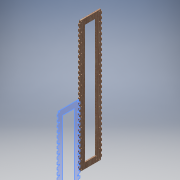
# Autodesk Inventor part: ArmTo
Saved by Autodesk Inventor 2019 (Build 230136000, 136)
## iProperties
Created: 2019-01-14
Part Number: ArmTo
Material: Wood (Birch)
Document SubType Name: Modeling
Designer: nxgam
Density: 0.55 g/cm^3
Appearance: Birch - Natural Polished
Author: nxgam
Autodesk Inventor part; units mm, degrees
ref_plane "YZ Plane" through (0, 0, 0) normal (1, 0, 0) x (0, 1, 0)
ref_plane "XZ Plane" through (0, 0, 0) normal (0, 1, 0) x (-1, 0, 0)
ref_plane "XY Plane" through (0, 0, 0) normal (0, 0, 1) x (1, 0, 0)
sketch "Sketch1" plane through (0, 0, 0) normal (1, 0, 0) x (0, 1, 0)
  line L0 (0, 50.8) -> (579.12, 50.8)
  line L1 (579.12, 50.8) -> (579.12, -50.8)
  line L2 (579.12, -50.8) -> (0, -50.8)
  line L3 (0, -50.8) -> (0, 50.8)
  point P0 (0, 0)
  point P1 (0, 0)
  dimension "d0" = 579.12
  dimension "d1" = 101.6
  constraints: 8 end point, 2 parallel, 1 coincident, 1 horizontal, 1 midpoint, 1 perpendicular, 1 other
  measures "d0" distance of L1.end L2.end
  measures "d1" distance of L0.end L1.end
extrude "Extrusion1" add sketch "Sketch1" along normal blind 5.08
sketch "Sketch2" plane through (5.08, 0, 0) normal (1, 0, 0) x (0, 0, -1)
  line L0 (-50.8, 579.12) -> (-50.8, 0) projected
  line L1 (-50.8, 0) -> (50.8, 0) projected
  line L2 (50.8, 0) -> (50.8, 579.12) projected
  line L3 (50.8, 579.12) -> (-50.8, 579.12) projected
  line L4 (-25.4, 553.72) -> (-25.4, 25.4)
  line L5 (-25.4, 25.4) -> (25.4, 25.4)
  line L6 (25.4, 25.4) -> (25.4, 553.72)
  line L7 (25.4, 553.72) -> (-25.4, 553.72)
  point P0 (0, 0)
  dimension "d4" = 50.8
  constraints: 8 end point, 3 other
  measures "d4" distance between parallel lines of L4 L6
extrude "Extrusion2" cut sketch "Sketch2" against normal blind 5.08 contours L7 L6 L5 L4
sketch "Sketch3" plane through (5.08, 0, 0) normal (1, 0, 0) x (0, 0, -1)
  circle A0 centre (-40.64, 45.72) radius 2 projected
  circle A1 centre (40.64, 5.08) radius 2 projected
  circle A2 centre (-40.64, 5.08) radius 2 projected
  circle A3 centre (40.64, 45.72) radius 2 projected
  line L0 (-42.545, 0) -> (42.545, 0) projected
  line L1 (45.72, 3.175) -> (45.72, 62.865) projected
  line L2 (42.545, 66.04) -> (38.735, 66.04) projected
  line L3 (35.56, 62.865) -> (35.56, 10.16) projected
  line L4 (35.56, 10.16) -> (-35.56, 10.16) projected
  line L5 (-35.56, 10.16) -> (-35.56, 62.865) projected
  line L6 (-38.735, 66.04) -> (-42.545, 66.04) projected
  line L7 (-45.72, 62.865) -> (-45.72, 3.175) projected
  arc A4 (-45.72, 3.175) -> (-42.545, 0) centre (-42.545, 3.175) ccw projected
  arc A5 (42.545, 0) -> (45.72, 3.175) centre (42.545, 3.175) ccw projected
  arc A6 (45.72, 62.865) -> (42.545, 66.04) centre (42.545, 62.865) ccw projected
  arc A7 (38.735, 66.04) -> (35.56, 62.865) centre (38.735, 62.865) ccw projected
  arc A8 (-35.56, 62.865) -> (-38.735, 66.04) centre (-38.735, 62.865) ccw projected
  arc A9 (-42.545, 66.04) -> (-45.72, 62.865) centre (-42.545, 62.865) ccw projected
  point P0 (0, 0)
  point P1 (-40.64, 45.72)
  point P2 (40.64, 5.08)
  point P3 (40.64, 45.72)
  point P4 (-40.64, 86.36)
  point P5 (40.64, 86.36)
  point P6 (-40.64, 127)
  point P7 (40.64, 127)
  point P8 (-40.64, 167.64)
  point P9 (40.64, 167.64)
  point P10 (-40.64, 208.28)
  point P11 (40.64, 208.28)
  point P12 (-40.64, 248.92)
  point P13 (40.64, 248.92)
  point P14 (-40.64, 289.56)
  point P15 (40.64, 289.56)
  point P16 (-40.64, 330.2)
  point P17 (40.64, 330.2)
  point P18 (-40.64, 370.84)
  point P19 (40.64, 370.84)
  point P20 (-40.64, 411.48)
  point P21 (40.64, 411.48)
  point P22 (-40.64, 452.12)
  point P23 (40.64, 452.12)
  point P24 (-40.64, 492.76)
  point P25 (40.64, 492.76)
  point P26 (-40.64, 533.4)
  point P27 (40.64, 533.4)
  point P28 (-40.64, 574.04)
  point P29 (40.64, 574.04)
  dimension "d9" = 40.64
  constraints: 4 coincident, 1 vertical, 26 other
  measures "d9" distance of point (-40.64, 45.72) point (-40.64, 86.36)
hole "Hole1" at (5.08, 5.08, 40.64) at (5.08, 45.72, 40.64) at (5.08, 5.08, -40.64) at (5.08, 45.72, -40.64) at (5.08, 86.36, 40.64) at (5.08, 86.36, -40.64) at (5.08, 127, 40.64) at (5.08, 127, -40.64) at (5.08, 167.64, 40.64) at (5.08, 167.64, -40.64) at (5.08, 208.28, 40.64) at (5.08, 208.28, -40.64) at (5.08, 248.92, 40.64) at (5.08, 248.92, -40.64) at (5.08, 289.56, 40.64) at (5.08, 289.56, -40.64) at (5.08, 330.2, 40.64) at (5.08, 330.2, -40.64) at (5.08, 370.84, 40.64) at (5.08, 370.84, -40.64) at (5.08, 411.48, 40.64) at (5.08, 411.48, -40.64) at (5.08, 452.12, 40.64) at (5.08, 452.12, -40.64) at (5.08, 492.76, 40.64) at (5.08, 492.76, -40.64) at (5.08, 533.4, 40.64) at (5.08, 533.4, -40.64) at (5.08, 574.04, 40.64) at (5.08, 574.04, -40.64) direction (-1, 0, 0) diameter 4 end through all
sketch "Sketch5" plane through (5.08, 0, 0) normal (1, 0, 0) x (0, 0, -1)
  circle A0 centre (-40.64, 574.04) radius 2 projected
  circle A1 centre (-40.64, 533.4) radius 2 projected
  circle A2 centre (-40.64, 492.76) radius 2 projected
  circle A3 centre (-40.64, 452.12) radius 2 projected
  circle A4 centre (-40.64, 411.48) radius 2 projected
  circle A5 centre (-40.64, 370.84) radius 2 projected
  circle A6 centre (-40.64, 330.2) radius 2 projected
  circle A7 centre (-40.64, 289.56) radius 2 projected
  circle A8 centre (-40.64, 248.92) radius 2 projected
  circle A9 centre (-40.64, 208.28) radius 2 projected
  circle A10 centre (-40.64, 167.64) radius 2 projected
  circle A11 centre (-40.64, 127) radius 2 projected
  circle A12 centre (-40.64, 86.36) radius 2 projected
  circle A13 centre (40.64, 5.08) radius 2 projected
  circle A14 centre (-40.64, 5.08) radius 2 projected
  circle A15 centre (-40.64, 45.72) radius 2 projected
  circle A16 centre (40.64, 45.72) radius 2 projected
  circle A17 centre (40.64, 86.36) radius 2 projected
  circle A18 centre (40.64, 127) radius 2 projected
  circle A19 centre (40.64, 167.64) radius 2 projected
  circle A20 centre (40.64, 208.28) radius 2 projected
  circle A21 centre (40.64, 248.92) radius 2 projected
  circle A22 centre (40.64, 289.56) radius 2 projected
  circle A23 centre (40.64, 330.2) radius 2 projected
  circle A24 centre (40.64, 370.84) radius 2 projected
  circle A25 centre (40.64, 411.48) radius 2 projected
  circle A26 centre (40.64, 452.12) radius 2 projected
  circle A27 centre (40.64, 492.76) radius 2 projected
  circle A28 centre (40.64, 533.4) radius 2 projected
  circle A29 centre (40.64, 574.04) radius 2 projected
  line L0 (25.4, 25.4) -> (-25.4, 25.4) projected
  line L1 (-25.4, 25.4) -> (-25.4, 553.72) projected
  line L2 (-25.4, 553.72) -> (25.4, 553.72) projected
  line L3 (25.4, 553.72) -> (25.4, 25.4) projected
  line L4 (-50.8, 579.12) -> (-50.8, 0) projected
  line L5 (-50.8, 0) -> (50.8, 0) projected
  line L6 (50.8, 0) -> (50.8, 579.12) projected
  line L7 (50.8, 579.12) -> (-50.8, 579.12) projected
  line L8 (-50.8, 579.12) -> (-45.72, 579.12)
  line L9 (-45.72, 579.12) -> (-45.72, 568.96)
  line L10 (-45.72, 568.96) -> (-50.8, 568.96)
  line L11 (-50.8, 568.96) -> (-50.8, 579.12)
  line L12 (-45.72, 558.8) -> (-45.72, 548.64)
  line L13 (-50.8, 548.64) -> (-50.8, 558.8)
  line L14 (-45.72, 548.64) -> (-50.8, 548.64)
  line L15 (-50.8, 558.8) -> (-45.72, 558.8)
  line L16 (-45.72, 538.48) -> (-45.72, 528.32)
  line L17 (-50.8, 528.32) -> (-50.8, 538.48)
  line L18 (-45.72, 528.32) -> (-50.8, 528.32)
  line L19 (-50.8, 538.48) -> (-45.72, 538.48)
  line L20 (-45.72, 518.16) -> (-45.72, 508)
  line L21 (-50.8, 508) -> (-50.8, 518.16)
  line L22 (-45.72, 508) -> (-50.8, 508)
  line L23 (-50.8, 518.16) -> (-45.72, 518.16)
  line L24 (-45.72, 497.84) -> (-45.72, 487.68)
  line L25 (-50.8, 487.68) -> (-50.8, 497.84)
  line L26 (-45.72, 487.68) -> (-50.8, 487.68)
  line L27 (-50.8, 497.84) -> (-45.72, 497.84)
  line L28 (-45.72, 477.52) -> (-45.72, 467.36)
  line L29 (-50.8, 467.36) -> (-50.8, 477.52)
  line L30 (-45.72, 467.36) -> (-50.8, 467.36)
  line L31 (-50.8, 477.52) -> (-45.72, 477.52)
  line L32 (-45.72, 457.2) -> (-45.72, 447.04)
  line L33 (-50.8, 447.04) -> (-50.8, 457.2)
  line L34 (-45.72, 447.04) -> (-50.8, 447.04)
  line L35 (-50.8, 457.2) -> (-45.72, 457.2)
  line L36 (-45.72, 436.88) -> (-45.72, 426.72)
  line L37 (-50.8, 426.72) -> (-50.8, 436.88)
  line L38 (-45.72, 426.72) -> (-50.8, 426.72)
  line L39 (-50.8, 436.88) -> (-45.72, 436.88)
  line L40 (-45.72, 416.56) -> (-45.72, 406.4)
  line L41 (-50.8, 406.4) -> (-50.8, 416.56)
  line L42 (-45.72, 406.4) -> (-50.8, 406.4)
  line L43 (-50.8, 416.56) -> (-45.72, 416.56)
  line L44 (-45.72, 396.24) -> (-45.72, 386.08)
  line L45 (-50.8, 386.08) -> (-50.8, 396.24)
  line L46 (-45.72, 386.08) -> (-50.8, 386.08)
  line L47 (-50.8, 396.24) -> (-45.72, 396.24)
  line L48 (-45.72, 375.92) -> (-45.72, 365.76)
  line L49 (-50.8, 365.76) -> (-50.8, 375.92)
  line L50 (-45.72, 365.76) -> (-50.8, 365.76)
  line L51 (-50.8, 375.92) -> (-45.72, 375.92)
  line L52 (-45.72, 355.6) -> (-45.72, 345.44)
  line L53 (-50.8, 345.44) -> (-50.8, 355.6)
  line L54 (-45.72, 345.44) -> (-50.8, 345.44)
  line L55 (-50.8, 355.6) -> (-45.72, 355.6)
  line L56 (-45.72, 335.28) -> (-45.72, 325.12)
  line L57 (-50.8, 325.12) -> (-50.8, 335.28)
  line L58 (-45.72, 325.12) -> (-50.8, 325.12)
  line L59 (-50.8, 335.28) -> (-45.72, 335.28)
  line L60 (-45.72, 314.96) -> (-45.72, 304.8)
  line L61 (-50.8, 304.8) -> (-50.8, 314.96)
  line L62 (-45.72, 304.8) -> (-50.8, 304.8)
  line L63 (-50.8, 314.96) -> (-45.72, 314.96)
  line L64 (-45.72, 294.64) -> (-45.72, 284.48)
  line L65 (-50.8, 284.48) -> (-50.8, 294.64)
  line L66 (-45.72, 284.48) -> (-50.8, 284.48)
  line L67 (-50.8, 294.64) -> (-45.72, 294.64)
  line L68 (-45.72, 274.32) -> (-45.72, 264.16)
  line L69 (-50.8, 264.16) -> (-50.8, 274.32)
  line L70 (-45.72, 264.16) -> (-50.8, 264.16)
  line L71 (-50.8, 274.32) -> (-45.72, 274.32)
  line L72 (-45.72, 254) -> (-45.72, 243.84)
  line L73 (-50.8, 243.84) -> (-50.8, 254)
  line L74 (-45.72, 243.84) -> (-50.8, 243.84)
  line L75 (-50.8, 254) -> (-45.72, 254)
  line L76 (-45.72, 233.68) -> (-45.72, 223.52)
  line L77 (-50.8, 223.52) -> (-50.8, 233.68)
  line L78 (-45.72, 223.52) -> (-50.8, 223.52)
  line L79 (-50.8, 233.68) -> (-45.72, 233.68)
  line L80 (-45.72, 213.36) -> (-45.72, 203.2)
  line L81 (-50.8, 203.2) -> (-50.8, 213.36)
  line L82 (-45.72, 203.2) -> (-50.8, 203.2)
  line L83 (-50.8, 213.36) -> (-45.72, 213.36)
  line L84 (-45.72, 193.04) -> (-45.72, 182.88)
  line L85 (-50.8, 182.88) -> (-50.8, 193.04)
  line L86 (-45.72, 182.88) -> (-50.8, 182.88)
  line L87 (-50.8, 193.04) -> (-45.72, 193.04)
  line L88 (-45.72, 172.72) -> (-45.72, 162.56)
  line L89 (-50.8, 162.56) -> (-50.8, 172.72)
  line L90 (-45.72, 162.56) -> (-50.8, 162.56)
  line L91 (-50.8, 172.72) -> (-45.72, 172.72)
  line L92 (-45.72, 152.4) -> (-45.72, 142.24)
  line L93 (-50.8, 142.24) -> (-50.8, 152.4)
  line L94 (-45.72, 142.24) -> (-50.8, 142.24)
  line L95 (-50.8, 152.4) -> (-45.72, 152.4)
  line L96 (-45.72, 132.08) -> (-45.72, 121.92)
  line L97 (-50.8, 121.92) -> (-50.8, 132.08)
  line L98 (-45.72, 121.92) -> (-50.8, 121.92)
  line L99 (-50.8, 132.08) -> (-45.72, 132.08)
  line L100 (-45.72, 111.76) -> (-45.72, 101.6)
  line L101 (-50.8, 101.6) -> (-50.8, 111.76)
  line L102 (-45.72, 101.6) -> (-50.8, 101.6)
  line L103 (-50.8, 111.76) -> (-45.72, 111.76)
  line L104 (-45.72, 91.44) -> (-45.72, 81.28)
  line L105 (-50.8, 81.28) -> (-50.8, 91.44)
  line L106 (-45.72, 81.28) -> (-50.8, 81.28)
  line L107 (-50.8, 91.44) -> (-45.72, 91.44)
  line L108 (-45.72, 71.12) -> (-45.72, 60.96)
  line L109 (-50.8, 60.96) -> (-50.8, 71.12)
  line L110 (-45.72, 60.96) -> (-50.8, 60.96)
  line L111 (-50.8, 71.12) -> (-45.72, 71.12)
  line L112 (-45.72, 50.8) -> (-45.72, 40.64)
  line L113 (-50.8, 40.64) -> (-50.8, 50.8)
  line L114 (-45.72, 40.64) -> (-50.8, 40.64)
  line L115 (-50.8, 50.8) -> (-45.72, 50.8)
  line L116 (-45.72, 30.48) -> (-45.72, 20.32)
  line L117 (-50.8, 20.32) -> (-50.8, 30.48)
  line L118 (-45.72, 20.32) -> (-50.8, 20.32)
  line L119 (-50.8, 30.48) -> (-45.72, 30.48)
  line L120 (-45.72, 10.16) -> (-45.72, 0)
  line L121 (-50.8, 0) -> (-50.8, 10.16)
  line L122 (-45.72, 0) -> (-50.8, 0)
  line L123 (-50.8, 10.16) -> (-45.72, 10.16)
  line L124 (-45.72, -10.16) -> (-45.72, -20.32)
  line L125 (-50.8, -20.32) -> (-50.8, -10.16)
  line L126 (-45.72, -20.32) -> (-50.8, -20.32)
  line L127 (-50.8, -10.16) -> (-45.72, -10.16)
  line L128 (0, 0) -> (0, 579.12) construction
  line L129 (50.8, 579.12) -> (-50.8, 579.12) construction
  line L130 (50.8, 579.12) -> (50.8, 0)
  line L131 (50.8, 579.12) -> (45.72, 579.12)
  line L132 (45.72, 579.12) -> (45.72, 568.96)
  line L133 (45.72, 568.96) -> (50.8, 568.96)
  line L134 (50.8, 568.96) -> (50.8, 579.12)
  line L135 (45.72, 558.8) -> (45.72, 548.64)
  line L136 (50.8, 548.64) -> (50.8, 558.8)
  line L137 (45.72, 548.64) -> (50.8, 548.64)
  line L138 (50.8, 558.8) -> (45.72, 558.8)
  line L139 (45.72, 538.48) -> (45.72, 528.32)
  line L140 (50.8, 528.32) -> (50.8, 538.48)
  line L141 (45.72, 528.32) -> (50.8, 528.32)
  line L142 (50.8, 538.48) -> (45.72, 538.48)
  line L143 (45.72, 518.16) -> (45.72, 508)
  line L144 (50.8, 508) -> (50.8, 518.16)
  line L145 (45.72, 508) -> (50.8, 508)
  line L146 (50.8, 518.16) -> (45.72, 518.16)
  line L147 (45.72, 497.84) -> (45.72, 487.68)
  line L148 (50.8, 487.68) -> (50.8, 497.84)
  line L149 (45.72, 487.68) -> (50.8, 487.68)
  line L150 (50.8, 497.84) -> (45.72, 497.84)
  line L151 (45.72, 477.52) -> (45.72, 467.36)
  line L152 (50.8, 467.36) -> (50.8, 477.52)
  line L153 (45.72, 467.36) -> (50.8, 467.36)
  line L154 (50.8, 477.52) -> (45.72, 477.52)
  line L155 (45.72, 457.2) -> (45.72, 447.04)
  line L156 (50.8, 447.04) -> (50.8, 457.2)
  line L157 (45.72, 447.04) -> (50.8, 447.04)
  line L158 (50.8, 457.2) -> (45.72, 457.2)
  line L159 (45.72, 436.88) -> (45.72, 426.72)
  line L160 (50.8, 426.72) -> (50.8, 436.88)
  line L161 (45.72, 426.72) -> (50.8, 426.72)
  line L162 (50.8, 436.88) -> (45.72, 436.88)
  line L163 (45.72, 416.56) -> (45.72, 406.4)
  line L164 (50.8, 406.4) -> (50.8, 416.56)
  line L165 (45.72, 406.4) -> (50.8, 406.4)
  line L166 (50.8, 416.56) -> (45.72, 416.56)
  line L167 (45.72, 396.24) -> (45.72, 386.08)
  line L168 (50.8, 386.08) -> (50.8, 396.24)
  line L169 (45.72, 386.08) -> (50.8, 386.08)
  line L170 (50.8, 396.24) -> (45.72, 396.24)
  line L171 (45.72, 375.92) -> (45.72, 365.76)
  line L172 (50.8, 365.76) -> (50.8, 375.92)
  line L173 (45.72, 365.76) -> (50.8, 365.76)
  line L174 (50.8, 375.92) -> (45.72, 375.92)
  line L175 (45.72, 355.6) -> (45.72, 345.44)
  line L176 (50.8, 345.44) -> (50.8, 355.6)
  line L177 (45.72, 345.44) -> (50.8, 345.44)
  line L178 (50.8, 355.6) -> (45.72, 355.6)
  line L179 (45.72, 335.28) -> (45.72, 325.12)
  line L180 (50.8, 325.12) -> (50.8, 335.28)
  line L181 (45.72, 325.12) -> (50.8, 325.12)
  line L182 (50.8, 335.28) -> (45.72, 335.28)
  line L183 (45.72, 314.96) -> (45.72, 304.8)
  line L184 (50.8, 304.8) -> (50.8, 314.96)
  line L185 (45.72, 304.8) -> (50.8, 304.8)
  line L186 (50.8, 314.96) -> (45.72, 314.96)
  line L187 (45.72, 294.64) -> (45.72, 284.48)
  line L188 (50.8, 284.48) -> (50.8, 294.64)
  line L189 (45.72, 284.48) -> (50.8, 284.48)
  line L190 (50.8, 294.64) -> (45.72, 294.64)
  line L191 (45.72, 274.32) -> (45.72, 264.16)
  line L192 (50.8, 264.16) -> (50.8, 274.32)
  line L193 (45.72, 264.16) -> (50.8, 264.16)
  line L194 (50.8, 274.32) -> (45.72, 274.32)
  line L195 (45.72, 254) -> (45.72, 243.84)
  line L196 (50.8, 243.84) -> (50.8, 254)
  line L197 (45.72, 243.84) -> (50.8, 243.84)
  line L198 (50.8, 254) -> (45.72, 254)
  line L199 (45.72, 233.68) -> (45.72, 223.52)
  line L200 (50.8, 223.52) -> (50.8, 233.68)
  line L201 (45.72, 223.52) -> (50.8, 223.52)
  line L202 (50.8, 233.68) -> (45.72, 233.68)
  line L203 (45.72, 213.36) -> (45.72, 203.2)
  line L204 (50.8, 203.2) -> (50.8, 213.36)
  line L205 (45.72, 203.2) -> (50.8, 203.2)
  line L206 (50.8, 213.36) -> (45.72, 213.36)
  line L207 (45.72, 193.04) -> (45.72, 182.88)
  line L208 (50.8, 182.88) -> (50.8, 193.04)
  line L209 (45.72, 182.88) -> (50.8, 182.88)
  line L210 (50.8, 193.04) -> (45.72, 193.04)
  line L211 (45.72, 172.72) -> (45.72, 162.56)
  line L212 (50.8, 162.56) -> (50.8, 172.72)
  line L213 (45.72, 162.56) -> (50.8, 162.56)
  line L214 (50.8, 172.72) -> (45.72, 172.72)
  line L215 (45.72, 152.4) -> (45.72, 142.24)
  line L216 (50.8, 142.24) -> (50.8, 152.4)
  line L217 (45.72, 142.24) -> (50.8, 142.24)
  line L218 (50.8, 152.4) -> (45.72, 152.4)
  line L219 (45.72, 132.08) -> (45.72, 121.92)
  line L220 (50.8, 121.92) -> (50.8, 132.08)
  line L221 (45.72, 121.92) -> (50.8, 121.92)
  line L222 (50.8, 132.08) -> (45.72, 132.08)
  line L223 (45.72, 111.76) -> (45.72, 101.6)
  line L224 (50.8, 101.6) -> (50.8, 111.76)
  line L225 (45.72, 101.6) -> (50.8, 101.6)
  line L226 (50.8, 111.76) -> (45.72, 111.76)
  line L227 (45.72, 91.44) -> (45.72, 81.28)
  line L228 (50.8, 81.28) -> (50.8, 91.44)
  line L229 (45.72, 81.28) -> (50.8, 81.28)
  line L230 (50.8, 91.44) -> (45.72, 91.44)
  line L231 (45.72, 71.12) -> (45.72, 60.96)
  line L232 (50.8, 60.96) -> (50.8, 71.12)
  line L233 (45.72, 60.96) -> (50.8, 60.96)
  line L234 (50.8, 71.12) -> (45.72, 71.12)
  line L235 (45.72, 50.8) -> (45.72, 40.64)
  line L236 (50.8, 40.64) -> (50.8, 50.8)
  line L237 (45.72, 40.64) -> (50.8, 40.64)
  line L238 (50.8, 50.8) -> (45.72, 50.8)
  line L239 (45.72, 30.48) -> (45.72, 20.32)
  line L240 (50.8, 20.32) -> (50.8, 30.48)
  line L241 (45.72, 20.32) -> (50.8, 20.32)
  line L242 (50.8, 30.48) -> (45.72, 30.48)
  line L243 (45.72, 10.16) -> (45.72, 0)
  line L244 (50.8, 0) -> (50.8, 10.16)
  line L245 (45.72, 0) -> (50.8, 0)
  line L246 (50.8, 10.16) -> (45.72, 10.16)
  line L247 (45.72, -10.16) -> (45.72, -20.32)
  line L248 (50.8, -20.32) -> (50.8, -10.16)
  line L249 (45.72, -20.32) -> (50.8, -20.32)
  line L250 (50.8, -10.16) -> (45.72, -10.16)
  dimension "d21" = 5.08
  dimension "d22" = 10.16
  dimension "d25" = 20.32
  constraints: 484 end point, 120 symmetric about line, 2 parallel, 1 horizontal, 1 midpoint, 1 perpendicular, 1 vertical, 232 other
  measures "d21" distance of L9.end L10.end
  measures "d22" distance of L8.end L9.end
  measures "d25" distance of L4.start L13.end
extrude "Extrusion3" cut sketch "Sketch5" against normal blind 25.4 contours L10 L9 L7 L132 L133 L6 L138 L135 L137 L142 L139 L141 L146 L143 L145 L150 L147 L149 L154 L151 L153 L158 L155 L157 L162 L159 L161 L166 L163 L165 L170 L167 L169 L174 L171 L173 L178 L175 L177 L182 L179 L181 L186 L183 L185 L190 L187 L189 L194 L191 L193 L198 L195 L197 L202 L199 L201 L206 L203 L205 L210 L207 L209 L214 L211 L213 L218 L215 L217 L222 L219 L221 L226 L223 L225 L230 L227 L229 L234 L231 L233 L238 L235 L237 L242 L239 L241 L246 L243 L5 L120 L123 L4 L118 L116 L119 L114 L112 L115 L110 L108 L111 L106 L104 L107 L102 L100 L103 L98 L96 L99 L94 L92 L95 L90 L88 L91 L86 L84 L87 L82 L80 L83 L78 L76 L79 L74 L72 L75 L70 L68 L71 L66 L64 L67 L62 L60 L63 L58 L56 L59 L54 L52 L55 L50 L48 L51 L46 L44 L47 L42 L40 L43 L38 L36 L39 L34 L32 L35 L30 L28 L31 L26 L24 L27 L22 L20 L23 L18 L16 L19 L14 L12 L15 keep common part
sketch "Sketch6" plane through (5.08, 0, 0) normal (1, 0, 0) x (0, 0, -1)
  line L0 (29.718, 20.1507) -> (26.924, 20.1507)
  line L1 (26.924, 14.9013) -> (26.924, 20.1507)
  line L2 (26.924, 9.652) -> (26.924, 14.9013)
  line L3 (26.924, 5.842) -> (26.924, 9.652)
  line L4 (29.718, 5.842) -> (26.924, 5.842)
  line L5 (29.718, 9.652) -> (29.718, 5.842)
  line L6 (29.718, 9.652) -> (26.924, 9.652)
  line L7 (29.718, 20.1507) -> (29.718, 14.9013)
  line L8 (29.718, 25.4) -> (29.718, 20.1507)
  line L9 (26.924, 25.4) -> (29.718, 25.4)
  line L10 (26.924, 25.4) -> (26.924, 29.21)
  line L11 (26.924, 29.21) -> (29.718, 29.21)
  line L12 (29.718, 29.21) -> (29.718, 25.4)
  line L13 (26.924, 20.1507) -> (26.924, 25.4)
  line L14 (26.924, 14.9013) -> (29.718, 14.9013)
  line L15 (29.718, 14.9013) -> (29.718, 9.652)
  point P0 (0, 0)
  constraints: 32 end point, 10 vertical, 6 horizontal, 12 other
extrude "Extrusion4" cut sketch "Sketch6" against normal blind 25.4 contours L0 L13 L9 L8 | L15 L6 L2 L14
equation "\"d25\" = 2 * d22"
body "Solid1"
